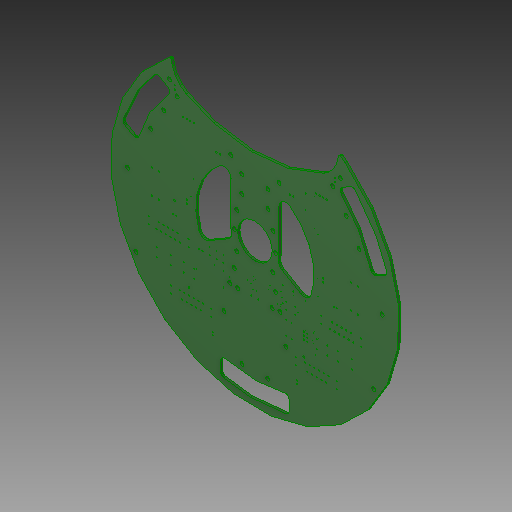
# Autodesk Inventor part: Board 1.brd_Outline
Saved by Autodesk Inventor 2017 (Build 210142000, 142)
## iProperties
Created: 2019-06-13
Part Number: Board 1.brd_Outline
Material: Generic
Document SubType Name: Modeling
Designer: Marc
Density: 1 g/cm^3
Appearance: Board Outline
Author: Marc
Autodesk Inventor part; units mm, degrees
ref_plane "YZ Plane" through (0, 0, 0) normal (1, 0, 0) x (0, 1, 0)
ref_plane "XZ Plane" through (0, 0, 0) normal (0, 1, 0) x (-1, 0, 0)
ref_plane "XY Plane" through (0, 0, 0) normal (0, 0, 1) x (1, 0, 0)
sketch "Sketch1" plane through (0, 0, 0) normal (0, 0, 1) x (1, 0, 0)
  line L0 (25.4618, 34.6584) -> (33.5639, 26.8882)
  line L1 (33.5639, 26.8882) -> (39.3789, 17.2857)
  line L2 (39.3789, 17.2857) -> (42.5104, 6.5054)
  line L3 (42.5104, 6.5054) -> (42.745, -4.7181)
  line L4 (42.745, -4.7181) -> (40.7535, -13.7294)
  line L5 (40.7535, -13.7294) -> (40.1788, -14.9013)
  line L6 (40.1788, -14.9013) -> (39.3204, -15.8846)
  line L7 (39.3204, -15.8846) -> (38.2368, -16.6122)
  line L8 (38.2368, -16.6122) -> (37.0018, -17.0345)
  line L9 (37.0018, -17.0345) -> (35.6995, -17.1228)
  line L10 (35.6995, -17.1228) -> (34.4188, -16.871)
  line L11 (34.4188, -16.871) -> (33.5153, -16.4628)
  line L12 (33.5153, -16.4628) -> (19.6223, -8.4417)
  line L13 (19.6223, -8.4417) -> (18.5867, -7.6472)
  line L14 (18.5867, -7.6472) -> (17.7922, -6.6117)
  line L15 (17.7922, -6.6117) -> (17.2926, -5.4058)
  line L16 (17.2926, -5.4058) -> (17.1222, -4.1118)
  line L17 (17.1222, -4.1118) -> (17.2066, -3.1972)
  line L18 (17.2066, -3.1972) -> (17.5017, 0.0028)
  line L19 (17.5017, 0.0028) -> (17.5017, 30.6288)
  line L20 (17.5017, 30.6288) -> (17.672, 31.923)
  line L21 (17.672, 31.923) -> (18.1716, 33.1289)
  line L22 (18.1716, 33.1289) -> (18.9662, 34.1644)
  line L23 (18.9662, 34.1644) -> (20.0017, 34.959)
  line L24 (20.0017, 34.959) -> (21.2077, 35.4585)
  line L25 (21.2077, 35.4585) -> (22.5018, 35.6288)
  line L26 (22.5018, 35.6288) -> (23.7959, 35.4584)
  line L27 (23.7959, 35.4584) -> (25.0018, 34.9589)
  line L28 (25.0018, 34.9589) -> (25.4618, 34.6584)
  line L29 (-19.6211, -8.4408) -> (-33.5098, -16.4596)
  line L30 (-33.5098, -16.4596) -> (-34.7157, -16.9591)
  line L31 (-34.7157, -16.9591) -> (-36.0099, -17.1294)
  line L32 (-36.0099, -17.1294) -> (-37.304, -16.959)
  line L33 (-37.304, -16.959) -> (-38.5099, -16.4595)
  line L34 (-38.5099, -16.4595) -> (-39.5454, -15.6649)
  line L35 (-39.5454, -15.6649) -> (-40.34, -14.6293)
  line L36 (-40.34, -14.6293) -> (-40.7482, -13.7257)
  line L37 (-40.7482, -13.7257) -> (-42.913, -2.7112)
  line L38 (-42.913, -2.7112) -> (-42.1534, 8.4883)
  line L39 (-42.1534, 8.4883) -> (-38.5209, 19.1096)
  line L40 (-38.5209, 19.1096) -> (-32.2633, 28.4289)
  line L41 (-32.2633, 28.4289) -> (-25.4611, 34.6541)
  line L42 (-25.4611, 34.6541) -> (-24.3174, 35.2831)
  line L43 (-24.3174, 35.2831) -> (-23.0499, 35.5947)
  line L44 (-23.0499, 35.5947) -> (-21.7449, 35.5676)
  line L45 (-21.7449, 35.5676) -> (-20.4914, 35.2037)
  line L46 (-20.4914, 35.2037) -> (-19.3748, 34.5278)
  line L47 (-19.3748, 34.5278) -> (-18.4712, 33.5858)
  line L48 (-18.4712, 33.5858) -> (-17.8421, 32.4421)
  line L49 (-17.8421, 32.4421) -> (-17.5306, 31.1746)
  line L50 (-17.5306, 31.1746) -> (-17.5003, 30.6251)
  line L51 (-17.5003, 30.6251) -> (-17.5003, 0.0028)
  line L52 (-17.5003, 0.0028) -> (-17.2054, -3.1967)
  line L53 (-17.2054, -3.1967) -> (-17.1363, -4.5002)
  line L54 (-17.1363, -4.5002) -> (-17.407, -5.7771)
  line L55 (-17.407, -5.7771) -> (-17.999, -6.9405)
  line L56 (-17.999, -6.9405) -> (-18.8719, -7.911)
  line L57 (-18.8719, -7.911) -> (-19.6211, -8.4408)
  line L58 (84.1395, 24.0165) -> (75.0573, 44.9741)
  line L59 (75.0573, 44.9741) -> (62.8687, 60.8586)
  line L60 (62.8687, 60.8586) -> (62.4021, 61.4876)
  line L61 (62.4021, 61.4876) -> (62.1142, 62.2159)
  line L62 (62.1142, 62.2159) -> (62.0246, 62.9939)
  line L63 (62.0246, 62.9939) -> (62.1395, 63.7686)
  line L64 (62.1395, 63.7686) -> (62.4509, 64.4872)
  line L65 (62.4509, 64.4872) -> (62.9376, 65.1007)
  line L66 (62.9376, 65.1007) -> (63.5243, 65.5433)
  line L67 (63.5243, 65.5433) -> (69.3163, 68.8873)
  line L68 (69.3163, 68.8873) -> (70.0399, 69.187)
  line L69 (70.0399, 69.187) -> (70.8163, 69.2892)
  line L70 (70.8163, 69.2892) -> (71.5928, 69.187)
  line L71 (71.5928, 69.187) -> (72.3163, 68.8873)
  line L72 (72.3163, 68.8873) -> (72.9377, 68.4105)
  line L73 (72.9377, 68.4105) -> (73.0065, 68.3394)
  line L74 (73.0065, 68.3394) -> (88.2054, 47.1172)
  line L75 (88.2054, 47.1172) -> (95.6867, 29.0554)
  line L76 (95.6867, 29.0554) -> (95.8144, 28.2827)
  line L77 (95.8144, 28.2827) -> (95.7379, 27.5033)
  line L78 (95.7379, 27.5033) -> (95.4622, 26.7703)
  line L79 (95.4622, 26.7703) -> (95.0062, 26.1336)
  line L80 (95.0062, 26.1336) -> (94.4009, 25.6366)
  line L81 (94.4009, 25.6366) -> (94.3161, 25.5857)
  line L82 (94.3161, 25.5857) -> (88.5243, 22.2418)
  line L83 (88.5243, 22.2418) -> (87.8008, 21.9421)
  line L84 (87.8008, 21.9421) -> (87.0243, 21.8399)
  line L85 (87.0243, 21.8399) -> (86.2479, 21.9421)
  line L86 (86.2479, 21.9421) -> (85.5243, 22.2418)
  line L87 (85.5243, 22.2418) -> (84.903, 22.7186)
  line L88 (84.903, 22.7186) -> (84.4262, 23.3399)
  line L89 (84.4262, 23.3399) -> (84.1395, 24.0165)
  line L90 (-88.5243, 22.2419) -> (-94.3156, 25.5855)
  line L91 (-94.3156, 25.5855) -> (-94.9369, 26.0622)
  line L92 (-94.9369, 26.0622) -> (-95.4137, 26.6835)
  line L93 (-95.4137, 26.6835) -> (-95.7134, 27.4071)
  line L94 (-95.7134, 27.4071) -> (-95.8156, 28.1836)
  line L95 (-95.8156, 28.1836) -> (-95.7134, 28.96)
  line L96 (-95.7134, 28.96) -> (-95.6862, 29.0552)
  line L97 (-95.6862, 29.0552) -> (-84.9072, 52.8291)
  line L98 (-84.9072, 52.8291) -> (-73.0061, 68.3392)
  line L99 (-73.0061, 68.3392) -> (-72.4008, 68.8362)
  line L100 (-72.4008, 68.8362) -> (-71.6876, 69.1597)
  line L101 (-71.6876, 69.1597) -> (-70.9149, 69.2874)
  line L102 (-70.9149, 69.2874) -> (-70.1354, 69.2109)
  line L103 (-70.1354, 69.2109) -> (-69.4024, 68.9352)
  line L104 (-69.4024, 68.9352) -> (-69.3159, 68.8872)
  line L105 (-69.3159, 68.8872) -> (-63.5242, 65.5432)
  line L106 (-63.5242, 65.5432) -> (-62.9029, 65.0665)
  line L107 (-62.9029, 65.0665) -> (-62.4262, 64.4452)
  line L108 (-62.4262, 64.4452) -> (-62.1265, 63.7216)
  line L109 (-62.1265, 63.7216) -> (-62.0242, 62.9452)
  line L110 (-62.0242, 62.9452) -> (-62.1265, 62.1687)
  line L111 (-62.1265, 62.1687) -> (-62.4262, 61.4452)
  line L112 (-62.4262, 61.4452) -> (-62.8687, 60.8586)
  line L113 (-62.8687, 60.8586) -> (-76.4774, 42.5144)
  line L114 (-76.4774, 42.5144) -> (-84.1395, 24.0165)
  line L115 (-84.1395, 24.0165) -> (-84.4509, 23.2979)
  line L116 (-84.4509, 23.2979) -> (-84.9377, 22.6845)
  line L117 (-84.9377, 22.6845) -> (-85.5667, 22.2179)
  line L118 (-85.5667, 22.2179) -> (-86.295, 21.9299)
  line L119 (-86.295, 21.9299) -> (-87.073, 21.8403)
  line L120 (-87.073, 21.8403) -> (-87.8477, 21.9552)
  line L121 (-87.8477, 21.9552) -> (-88.5243, 22.2419)
  line L122 (22.6786, -97.3937) -> (-3.2985, -99.9451)
  line L123 (-3.2985, -99.9451) -> (-22.6803, -97.3932)
  line L124 (-22.6803, -97.3932) -> (-23.4133, -97.1176)
  line L125 (-23.4133, -97.1176) -> (-24.05, -96.6616)
  line L126 (-24.05, -96.6616) -> (-24.547, -96.0563)
  line L127 (-24.547, -96.0563) -> (-24.8704, -95.3431)
  line L128 (-24.8704, -95.3431) -> (-24.9982, -94.5704)
  line L129 (-24.9982, -94.5704) -> (-24.9999, -94.4715)
  line L130 (-24.9999, -94.4715) -> (-24.9999, -87.7853)
  line L131 (-24.9999, -87.7853) -> (-24.8977, -87.0088)
  line L132 (-24.8977, -87.0088) -> (-24.598, -86.2853)
  line L133 (-24.598, -86.2853) -> (-24.1213, -85.664)
  line L134 (-24.1213, -85.664) -> (-23.5, -85.1872)
  line L135 (-23.5, -85.1872) -> (-22.7764, -84.8875)
  line L136 (-22.7764, -84.8875) -> (-22, -84.7853)
  line L137 (-22, -84.7853) -> (-21.2707, -84.8753)
  line L138 (-21.2707, -84.8753) -> (1.4192, -87.4888)
  line L139 (1.4192, -87.4888) -> (21.2691, -84.8757)
  line L140 (21.2691, -84.8757) -> (22.0471, -84.7861)
  line L141 (22.0471, -84.7861) -> (22.8217, -84.9009)
  line L142 (22.8217, -84.9009) -> (23.5403, -85.2123)
  line L143 (23.5403, -85.2123) -> (24.1538, -85.6991)
  line L144 (24.1538, -85.6991) -> (24.6204, -86.3281)
  line L145 (24.6204, -86.3281) -> (24.9083, -87.0564)
  line L146 (24.9083, -87.0564) -> (24.9983, -87.7857)
  line L147 (24.9983, -87.7857) -> (24.9983, -94.4719)
  line L148 (24.9983, -94.4719) -> (24.896, -95.2484)
  line L149 (24.896, -95.2484) -> (24.5963, -95.9719)
  line L150 (24.5963, -95.9719) -> (24.1195, -96.5932)
  line L151 (24.1195, -96.5932) -> (23.4982, -97.07)
  line L152 (23.4982, -97.07) -> (22.7746, -97.3697)
  line L153 (22.7746, -97.3697) -> (22.6786, -97.3937)
  line L154 (-60.7504, 83.7892) -> (-60.8105, 84.0432)
  line L155 (-60.8105, 84.0432) -> (-60.9343, 84.273)
  line L156 (-60.9343, 84.273) -> (-61.1134, 84.463)
  line L157 (-61.1134, 84.463) -> (-61.3355, 84.6001)
  line L158 (-61.3355, 84.6001) -> (-61.5856, 84.6751)
  line L159 (-61.5856, 84.6751) -> (-61.8465, 84.6827)
  line L160 (-61.8465, 84.6827) -> (-62.1005, 84.6226)
  line L161 (-62.1005, 84.6226) -> (-62.3303, 84.4988)
  line L162 (-62.3303, 84.4988) -> (-62.339, 84.4925)
  line L163 (-62.339, 84.4925) -> (-82.0829, 65.4791)
  line L164 (-82.0829, 65.4791) -> (-96.2331, 42.0034)
  line L165 (-96.2331, 42.0034) -> (-103.8251, 15.6653)
  line L166 (-103.8251, 15.6653) -> (-104.3417, -11.7403)
  line L167 (-104.3417, -11.7403) -> (-97.7475, -38.3458)
  line L168 (-97.7475, -38.3458) -> (-84.492, -62.338)
  line L169 (-84.492, -62.338) -> (-65.4786, -82.082)
  line L170 (-65.4786, -82.082) -> (-42.0029, -96.2321)
  line L171 (-42.0029, -96.2321) -> (-15.6648, -103.8242)
  line L172 (-15.6648, -103.8242) -> (11.7408, -104.3407)
  line L173 (11.7408, -104.3407) -> (38.3463, -97.7466)
  line L174 (38.3463, -97.7466) -> (62.3385, -84.4911)
  line L175 (62.3385, -84.4911) -> (82.0825, -65.4777)
  line L176 (82.0825, -65.4777) -> (96.2326, -42.002)
  line L177 (96.2326, -42.002) -> (103.8247, -15.6639)
  line L178 (103.8247, -15.6639) -> (104.3412, 11.7417)
  line L179 (104.3412, 11.7417) -> (97.7471, 38.3472)
  line L180 (97.7471, 38.3472) -> (84.4916, 62.3395)
  line L181 (84.4916, 62.3395) -> (65.4782, 82.0834)
  line L182 (65.4782, 82.0834) -> (62.338, 84.493)
  line L183 (62.338, 84.493) -> (62.1094, 84.6192)
  line L184 (62.1094, 84.6192) -> (61.8561, 84.682)
  line L185 (61.8561, 84.682) -> (61.5951, 84.6771)
  line L186 (61.5951, 84.6771) -> (61.3442, 84.6048)
  line L187 (61.3442, 84.6048) -> (61.1206, 84.47)
  line L188 (61.1206, 84.47) -> (60.9396, 84.282)
  line L189 (60.9396, 84.282) -> (60.8133, 84.0535)
  line L190 (60.8133, 84.0535) -> (60.7505, 83.8001)
  line L191 (60.7505, 83.8001) -> (60.7494, 83.7897)
  line L192 (60.7494, 83.7897) -> (59.5029, 78.5248)
  line L193 (59.5029, 78.5248) -> (56.9362, 73.7619)
  line L194 (56.9362, 73.7619) -> (53.2243, 69.8257)
  line L195 (53.2243, 69.8257) -> (50.001, 67.6671)
  line L196 (50.001, 67.6671) -> (24.4028, 57.8709)
  line L197 (24.4028, 57.8709) -> (-2.8586, 55.0339)
  line L198 (-2.8586, 55.0339) -> (-29.9254, 59.3493)
  line L199 (-29.9254, 59.3493) -> (-50.0022, 67.6648)
  line L200 (-50.0022, 67.6648) -> (-54.3828, 70.8409)
  line L201 (-54.3828, 70.8409) -> (-57.7921, 75.0425)
  line L202 (-57.7921, 75.0425) -> (-59.9977, 79.9833)
  line L203 (-59.9977, 79.9833) -> (-60.7504, 83.7892)
  line L204 (12.5, 0) -> (12.3931, 1.6316)
  line L205 (12.3931, 1.6316) -> (12.0741, 3.2352)
  line L206 (12.0741, 3.2352) -> (10.8253, 6.25)
  line L207 (10.8253, 6.25) -> (8.8388, 8.8388)
  line L208 (8.8388, 8.8388) -> (6.25, 10.8253)
  line L209 (6.25, 10.8253) -> (3.2352, 12.0741)
  line L210 (3.2352, 12.0741) -> (0, 12.5)
  line L211 (0, 12.5) -> (-3.2352, 12.0741)
  line L212 (-3.2352, 12.0741) -> (-6.25, 10.8253)
  line L213 (-6.25, 10.8253) -> (-8.8388, 8.8388)
  line L214 (-8.8388, 8.8388) -> (-10.8253, 6.25)
  line L215 (-10.8253, 6.25) -> (-12.0741, 3.2352)
  line L216 (-12.0741, 3.2352) -> (-12.5, 0)
  line L217 (-12.5, 0) -> (-12.0741, -3.2352)
  line L218 (-12.0741, -3.2352) -> (-10.8253, -6.25)
  line L219 (-10.8253, -6.25) -> (-8.8388, -8.8388)
  line L220 (-8.8388, -8.8388) -> (-6.25, -10.8253)
  line L221 (-6.25, -10.8253) -> (-3.2352, -12.0741)
  line L222 (-3.2352, -12.0741) -> (0, -12.5)
  line L223 (0, -12.5) -> (3.2352, -12.0741)
  line L224 (3.2352, -12.0741) -> (6.25, -10.8253)
  line L225 (6.25, -10.8253) -> (8.8388, -8.8388)
  line L226 (8.8388, -8.8388) -> (10.8253, -6.25)
  line L227 (10.8253, -6.25) -> (12.0741, -3.2352)
  line L228 (12.0741, -3.2352) -> (12.5, 0)
  circle A0 centre (-33.02, -25.4) radius 0.405
  circle A1 centre (-27.94, -25.4) radius 0.405
  circle A2 centre (-33.02, -20.32) radius 0.405
  circle A3 centre (-27.94, -20.32) radius 0.405
  circle A4 centre (2.54, -35.56) radius 0.405
  circle A5 centre (-2.54, -35.56) radius 0.405
  circle A6 centre (-74.93, 8.89) radius 0.51
  circle A7 centre (-69.85, 8.89) radius 0.51
  circle A8 centre (-59.44, -12.7) radius 0.405
  circle A9 centre (-57.4, -12.7) radius 0.405
  circle A10 centre (-77.09, -22.86) radius 0.405
  circle A11 centre (-77.09, -27.94) radius 0.405
  circle A12 centre (-48.26, -22.86) radius 0.405
  circle A13 centre (-48.26, -27.94) radius 0.405
  circle A14 centre (74.93, 8.89) radius 0.51
  circle A15 centre (69.85, 8.89) radius 0.51
  circle A16 centre (59.44, -12.7) radius 0.405
  circle A17 centre (57.4, -12.7) radius 0.405
  circle A18 centre (48.26, -22.86) radius 0.405
  circle A19 centre (48.26, -27.94) radius 0.405
  circle A20 centre (77.09, -22.86) radius 0.405
  circle A21 centre (77.09, -27.94) radius 0.405
  circle A22 centre (-74.93, -8.89) radius 0.51
  circle A23 centre (-69.85, -8.89) radius 0.51
  circle A24 centre (-30.48, -74.68) radius 0.405
  circle A25 centre (-30.48, -72.64) radius 0.405
  circle A26 centre (-31.75, -63.5) radius 0.405
  circle A27 centre (-31.75, -58.42) radius 0.405
  circle A28 centre (-60.96, -63.5) radius 0.405
  circle A29 centre (-60.96, -58.42) radius 0.405
  circle A30 centre (74.93, -8.89) radius 0.51
  circle A31 centre (69.85, -8.89) radius 0.51
  circle A32 centre (30.48, -74.68) radius 0.405
  circle A33 centre (30.48, -72.64) radius 0.405
  circle A34 centre (59.56, -63.5) radius 0.405
  circle A35 centre (59.56, -58.42) radius 0.405
  circle A36 centre (29.59, -63.5) radius 0.405
  circle A37 centre (29.59, -58.42) radius 0.405
  circle A38 centre (22.86, -31.75) radius 0.405
  circle A39 centre (22.86, -26.67) radius 0.405
  circle A40 centre (29.21, -31.75) radius 0.405
  circle A41 centre (29.21, -26.67) radius 0.405
  circle A42 centre (27.94, -17.78) radius 0.405
  circle A43 centre (20.32, -17.78) radius 0.405
  circle A44 centre (-44.07, -39.37) radius 0.405
  circle A45 centre (-51.69, -39.37) radius 0.405
  circle A46 centre (45.09, -39.37) radius 0.405
  circle A47 centre (52.71, -39.37) radius 0.405
  circle A48 centre (-44.2, -45.72) radius 0.405
  circle A49 centre (-51.82, -45.72) radius 0.405
  circle A50 centre (45.09, -45.72) radius 0.405
  circle A51 centre (52.71, -45.72) radius 0.405
  circle A52 centre (-44.45, 52.07) radius 0.51
  circle A53 centre (-46.99, 52.07) radius 0.51
  circle A54 centre (-49.53, 52.07) radius 0.51
  circle A55 centre (-52.07, 52.07) radius 0.51
  circle A56 centre (-49.53, 1.27) radius 0.51
  circle A57 centre (-49.53, -1.27) radius 0.51
  circle A58 centre (44.45, 52.07) radius 0.51
  circle A59 centre (46.99, 52.07) radius 0.51
  circle A60 centre (49.53, 52.07) radius 0.51
  circle A61 centre (52.07, 52.07) radius 0.51
  circle A62 centre (35.56, -39.37) radius 0.51
  circle A63 centre (38.1, -39.37) radius 0.51
  circle A64 centre (35.56, -41.91) radius 0.51
  circle A65 centre (38.1, -41.91) radius 0.51
  circle A66 centre (35.56, -44.45) radius 0.51
  circle A67 centre (38.1, -44.45) radius 0.51
  circle A68 centre (-58.29, 66.29) radius 0.51
  circle A69 centre (-58.29, 68.83) radius 0.51
  circle A70 centre (58.29, 66.29) radius 0.51
  circle A71 centre (58.29, 68.83) radius 0.51
  circle A72 centre (-27.94, 41.91) radius 0.51
  circle A73 centre (-25.4, 41.91) radius 0.51
  circle A74 centre (27.94, 41.91) radius 0.51
  circle A75 centre (25.4, 41.91) radius 0.51
  circle A76 centre (-40.64, -25.4) radius 0.51
  circle A77 centre (-38.1, -25.4) radius 0.51
  circle A78 centre (49.53, -1.27) radius 0.51
  circle A79 centre (49.53, 1.27) radius 0.51
  circle A80 centre (-71.58, -28.12) radius 0.51
  circle A81 centre (-69.88, -23.06) radius 0.51
  circle A82 centre (-68.18, -28.12) radius 0.51
  circle A83 centre (-66.48, -23.06) radius 0.51
  circle A84 centre (-64.78, -28.12) radius 0.51
  circle A85 centre (-63.07, -23.06) radius 0.51
  circle A86 centre (-61.37, -28.12) radius 0.51
  circle A87 centre (-59.67, -23.06) radius 0.51
  circle A88 centre (-57.97, -28.12) radius 0.51
  circle A89 centre (-56.27, -23.06) radius 0.51
  circle A90 centre (-54.57, -28.12) radius 0.51
  circle A91 centre (54.53, -28.12) radius 0.51
  circle A92 centre (56.23, -23.06) radius 0.51
  circle A93 centre (57.93, -28.12) radius 0.51
  circle A94 centre (59.63, -23.06) radius 0.51
  circle A95 centre (61.33, -28.12) radius 0.51
  circle A96 centre (63.04, -23.06) radius 0.51
  circle A97 centre (64.74, -28.12) radius 0.51
  circle A98 centre (66.44, -23.06) radius 0.51
  circle A99 centre (68.14, -28.12) radius 0.51
  circle A100 centre (69.84, -23.06) radius 0.51
  circle A101 centre (71.55, -28.12) radius 0.51
  circle A102 centre (-37.64, -58.24) radius 0.51
  circle A103 centre (-39.34, -63.3) radius 0.51
  circle A104 centre (-41.04, -58.24) radius 0.51
  circle A105 centre (-42.74, -63.3) radius 0.51
  circle A106 centre (-44.44, -58.24) radius 0.51
  circle A107 centre (-46.15, -63.3) radius 0.51
  circle A108 centre (-47.85, -58.24) radius 0.51
  circle A109 centre (-49.55, -63.3) radius 0.51
  circle A110 centre (-51.25, -58.24) radius 0.51
  circle A111 centre (-52.95, -63.3) radius 0.51
  circle A112 centre (-54.65, -58.24) radius 0.51
  circle A113 centre (53.42, -58.24) radius 0.51
  circle A114 centre (51.72, -63.3) radius 0.51
  circle A115 centre (50.02, -58.24) radius 0.51
  circle A116 centre (48.32, -63.3) radius 0.51
  circle A117 centre (46.62, -58.24) radius 0.51
  circle A118 centre (44.91, -63.3) radius 0.51
  circle A119 centre (43.21, -58.24) radius 0.51
  circle A120 centre (41.51, -63.3) radius 0.51
  circle A121 centre (39.81, -58.24) radius 0.51
  circle A122 centre (38.11, -63.3) radius 0.51
  circle A123 centre (36.4, -58.24) radius 0.51
  circle A124 centre (-22.86, -25.27) radius 0.405
  circle A125 centre (-22.86, -20.45) radius 0.405
  circle A126 centre (22.86, -38.1) radius 0.405
  circle A127 centre (22.86, -48.26) radius 0.405
  circle A128 centre (-61.34, -39.5) radius 0.405
  circle A129 centre (-71.5, -39.5) radius 0.405
  circle A130 centre (60.33, -39.37) radius 0.405
  circle A131 centre (70.48, -39.37) radius 0.405
  circle A132 centre (-61.21, -45.72) radius 0.405
  circle A133 centre (-71.37, -45.72) radius 0.405
  circle A134 centre (60.33, -45.72) radius 0.405
  circle A135 centre (70.48, -45.72) radius 0.405
  circle A136 centre (26.67, -48.26) radius 0.405
  circle A137 centre (26.67, -38.1) radius 0.405
  circle A138 centre (36.83, 48.26) radius 0.405
  circle A139 centre (36.83, 38.1) radius 0.405
  circle A140 centre (-22.86, -30.48) radius 0.405
  circle A141 centre (-22.86, -40.64) radius 0.405
  circle A142 centre (-62.1263, 70.7101) radius 1.5
  circle A143 centre (-56.586, 62.7977) radius 1.5
  circle A144 centre (56.5854, 62.7977) radius 1.5
  circle A145 centre (62.1257, 70.7101) radius 1.5
  circle A146 centre (-17.5004, 45.551) radius 1.5
  circle A147 centre (17.5016, 45.5511) radius 1.5
  circle A148 centre (-9.5, 37.4962) radius 1.5
  circle A149 centre (9.5, 37.4962) radius 1.5
  circle A150 centre (-9.5, 24.9962) radius 1.5
  circle A151 centre (9.5, 24.9962) radius 1.5
  circle A152 centre (-13.0815, 13.0815) radius 1.5
  circle A153 centre (13.0815, 13.0815) radius 1.5
  circle A154 centre (-15.0008, 0.0024) radius 1.5
  circle A155 centre (15.0008, 0.0024) radius 1.5
  circle A156 centre (-13.0815, -13.0815) radius 1.5
  circle A157 centre (13.0815, -13.0815) radius 1.5
  circle A158 centre (-15.0008, -24.507) radius 1.5
  circle A159 centre (15.0008, -24.507) radius 1.5
  circle A160 centre (-18.1774, -35.3844) radius 1.5
  circle A161 centre (-12.4968, -35.9326) radius 1.5
  circle A162 centre (12.4968, -35.9326) radius 1.5
  circle A163 centre (18.1774, -35.3844) radius 1.5
  circle A164 centre (-22.4968, -55.1826) radius 1.5
  circle A165 centre (22.4968, -55.1826) radius 1.5
  circle A166 centre (-9.375, -82.0001) radius 1.45
  circle A167 centre (9.3761, -81.9899) radius 1.45
  circle A168 centre (-86.5112, -49.9474) radius 1.5
  circle A169 centre (-92.4893, 0) radius 1.5
  circle A170 centre (-75.7016, 32.8809) radius 1.45
  circle A171 centre (-66.3188, 49.115) radius 1.45
  circle A172 centre (66.3266, 49.1189) radius 1.45
  circle A173 centre (75.6955, 32.8779) radius 1.45
  circle A174 centre (92.5005, 0) radius 1.5
  circle A175 centre (86.5112, -49.9474) radius 1.5
  circle A176 centre (-29.2608, -29.718) radius 0.3048
  circle A177 centre (0.9906, -31.0896) radius 0.3048
  circle A178 centre (-44.577, 16.764) radius 0.3048
  circle A179 centre (-47.8536, -53.2638) radius 0.6985
  circle A180 centre (35.5092, -55.3212) radius 0.6985
  circle A181 centre (10.0584, -25.7556) radius 0.175
  circle A182 centre (18.9738, -22.1742) radius 0.175
  circle A183 centre (43.5864, 29.4132) radius 0.175
  circle A184 centre (16.5354, -31.3944) radius 0.175
  circle A185 centre (45.2628, -0.762) radius 0.175
  circle A186 centre (19.1262, -30.4038) radius 0.175
  circle A187 centre (0.1524, -24.003) radius 0.175
  circle A188 centre (-1.2192, -22.86) radius 0.175
  circle A189 centre (42.3672, -36.6522) radius 0.175
  circle A190 centre (-0.8382, -25.4508) radius 0.175
  circle A191 centre (-18.288, -31.7754) radius 0.175
  circle A192 centre (-2.7432, -28.2702) radius 0.175
  circle A193 centre (-42.3672, -38.7096) radius 0.175
  circle A194 centre (36.7284, -37.8714) radius 0.175
  circle A195 centre (-5.4864, -27.2796) radius 0.175
  circle A196 centre (10.8204, -22.5552) radius 0.175
  circle A197 centre (41.7576, -41.529) radius 0.175
  circle A198 centre (44.0436, -49.7586) radius 0.175
  circle A199 centre (27.8892, -20.193) radius 0.175
  circle A200 centre (42.9768, -35.2806) radius 0.175
  circle A201 centre (45.8724, -38.1762) radius 0.175
  circle A202 centre (19.812, -25.6032) radius 0.175
  circle A203 centre (42.3672, -43.053) radius 0.175
  circle A204 centre (-1.3716, -31.0896) radius 0.3048
  circle A205 centre (20.3454, -29.0322) radius 0.3048
  circle A206 centre (31.242, -29.337) radius 0.3048
  circle A207 centre (-46.4058, 4.953) radius 0.3048
  circle A208 centre (18.9738, -32.004) radius 0.175
  circle A209 centre (36.6522, -19.2786) radius 0.175
  circle A210 centre (45.8724, -11.9634) radius 0.175
  circle A211 centre (45.8724, 27.1272) radius 0.175
  circle A212 centre (43.5864, 49.53) radius 0.175
  circle A213 centre (-58.42, -3.81) radius 0.6985
  constraints: 458 end point, 214 centre point
extrude "Board 1.brd_Outline" add sketch "Sketch1" along normal blind 1.6
body "Solid1"
